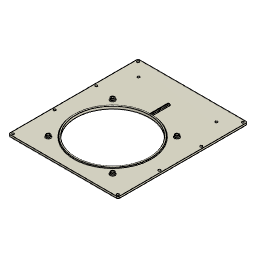
Lid - 120mm Fan (Autodesk Fusion 360 design; units mm, degrees)
Autodesk Fusion 360 part; units mm, degrees
imported_body "Derived Base Feature5" makes body 1
imported_body "Derived Base Feature6" makes body 2
imported_body "Derived Base Feature2" makes body 3
imported_body "Derived Base Feature3" makes body 4
imported_body "Derived Base Feature4" makes body 5
ref_plane "WorkPlane1" through (0, 0, 123.8) normal (0, 0, 1) x (1, 0, 0)
sketch "Sketch1" plane through (0, 0, 123.8) normal (0, 0, 1) x (1, 0, 0)
  circle A0 centre (-85.5, 170) radius 1.4 construction
  line L0 (-81.5, 4) -> (-81.5, 166) construction
  line L1 (-81.5, 166) -> (-81.5, 167) construction
  line L2 (-81.5, 167) -> (-77.5, 167) construction
  line L3 (-77.5, 167) -> (-77.5, 174) construction
  line L4 (-77.5, 174) -> (-81.5, 174) construction
  line L5 (-81.5, 174) -> (-86.5, 174) construction
  line L6 (-87.2574, 174) -> (-87.5, 174) construction
  line L7 (-87.5, 174) -> (-89.5, 172) construction
  line L8 (-89.5, 172) -> (-89.5, 0) construction
  line L9 (-89.5, 0) -> (-81.5, 0) construction
  line L10 (-81.5, 0) -> (-81.5, 4) construction
  circle A1 centre (85.5, 170) radius 1.4 construction
  line L11 (89.5, 0) -> (89.5, 172) construction
  line L12 (89.5, 172) -> (87.5, 174) construction
  line L13 (87.5, 174) -> (86.5, 174) construction
  line L14 (86.5, 174) -> (86.5, 177) construction
  line L15 (86.5, 177) -> (86.45, 177) construction
  line L16 (86.45, 177) -> (86.45, 174) construction
  line L17 (86.45, 174) -> (81.5, 174) construction
  line L18 (81.5, 174) -> (77.5, 174) construction
  line L19 (77.5, 174) -> (77.5, 167) construction
  line L20 (77.5, 167) -> (81.5, 167) construction
  line L21 (81.5, 167) -> (81.5, 0) construction
  line L22 (81.5, 0) -> (89.5, 0) construction
  line L23 (81.5, 0) -> (81.5, -37.7937) construction
  line L24 (81.5, -37.7937) -> (87.5, -37.7937) construction
  line L25 (87.5, -37.7937) -> (89.5, -35.7937) construction
  line L26 (89.5, -35.7937) -> (89.5, -5) construction
  line L27 (89.5, -5) -> (89.5, 0) construction
  line L28 (89.5, 0) -> (81.5, 0) construction
  line L29 (-89.5, 0) -> (-89.5, -35.7937) construction
  line L30 (-89.5, -35.7937) -> (-87.5, -37.7937) construction
  line L31 (-87.5, -37.7937) -> (-81.5, -37.7937) construction
  line L32 (-81.5, -37.7937) -> (-81.5, -5) construction
  line L33 (-81.5, -5) -> (-81.5, 0) construction
  line L34 (-81.5, 0) -> (-89.5, 0) construction
  line L35 (87.5, -37.7937) -> (-87.5, -37.7937) construction
  line L36 (-77.3, 174) -> (77.3, 174) construction
  line L37 (-77.5, 174) -> (77.5, 174)
  line L38 (77.5, 174) -> (87.5, 174)
  line L39 (87.5, 174) -> (89.5, 172)
  line L40 (89.5, 172) -> (89.5, -35.7937)
  line L41 (89.5, -35.7937) -> (87.5, -37.7937)
  line L42 (-87.5, -37.7937) -> (87.5, -37.7937)
  line L43 (-87.5, -37.7937) -> (-89.5, -35.7937)
  line L44 (-89.5, -35.7937) -> (-89.5, 172)
  line L45 (-89.5, 172) -> (-87.5, 174)
  line L46 (-87.5, 174) -> (-77.3, 174)
  circle A2 centre (-85.5, 170) radius 1.8
  circle A3 centre (-85.5, 102) radius 1.8
  circle A4 centre (-85.5, 34) radius 1.8
  circle A5 centre (-85.5, -34) radius 1.8
  circle A6 centre (85.5, -34) radius 1.8
  circle A7 centre (85.5, 34) radius 1.8
  circle A8 centre (85.5, 102) radius 1.8
  circle A9 centre (85.5, 170) radius 1.8
  circle A10 centre (-85.5, -34) radius 1.4 construction
  circle A11 centre (85.5, -34) radius 1.4 construction
  circle A12 centre (85.5, 34) radius 1.4 construction
  circle A13 centre (-85.5, 34) radius 1.4 construction
  circle A14 centre (85.5, 102) radius 1.4 construction
  circle A15 centre (-85.5, 102) radius 1.4 construction
  line L47 (-86.5, 174) -> (-87.2574, 174)
  line L48 (-77.5, 173.8) -> (-77.3, 173.8)
  line L49 (-77.3, 173.8) -> (77.5, 173.8)
  line L50 (77.5, 173.8) -> (87.4172, 173.8)
  line L51 (87.4172, 173.8) -> (89.3, 171.9172)
  line L52 (89.3, 171.9172) -> (89.3, -35.7109)
  line L53 (89.3, -35.7109) -> (87.4172, -37.5937)
  line L54 (-87.4172, -37.5937) -> (87.4172, -37.5937)
  line L55 (-87.4172, -37.5937) -> (-89.3, -35.7109)
  line L56 (-89.3, -35.7109) -> (-89.3, 171.9172)
  line L57 (-89.3, 171.9172) -> (-87.4172, 173.8)
  line L58 (-87.4172, 173.8) -> (-77.3, 173.8)
  dimension "d2" = 0.2
  dimension "d4" = 3.6
  dimension "d5" = 3.6
  dimension "d6" = 3.6
  dimension "d7" = 3.6
  dimension "d8" = 3.6
  dimension "d9" = 3.6
  dimension "d10" = 3.6
  dimension "d11" = 3.6
  constraint coincident L3.end L4.start
  constraint coincident L18.end L19.start
  constraint coincident L12.end L13.start
  constraint coincident L11.end L12.start
  constraint coincident L25.end L26.start
  constraint coincident L24.end L25.start
  constraint coincident L30.end L31.start
  constraint coincident L29.end L30.start
  constraint coincident L7.end L8.start
  constraint coincident L6.end L7.start
  constraint coincident L36.start L46.end
  constraint concentric A0 A2
  constraint concentric A1 A9
  constraint concentric A5 A10
  constraint concentric A6 A11
  constraint concentric A4 A13
  constraint concentric A7 A12
  constraint concentric A8 A14
  constraint concentric A3 A15
  measures "d4" diameter of A2
  measures "d5" diameter of A9
  measures "d6" diameter of A8
  measures "d7" diameter of A3
  measures "d8" diameter of A7
  measures "d9" diameter of A6
  measures "d10" diameter of A4
  measures "d11" diameter of A5
extrude "Extrude1" add sketch "Sketch1" along normal blind 3 separate body contours L48 L49 L50 L51 L52 L53 L54 L55 L56 L57 L58 makes body 6
ref_plane "WorkPlane2" through (-3.8893, 68.1031, 125.3) normal (1, 0, 0) x (0, 1, 0)
sketch "Sketch2" plane through (-3.8893, 68.1031, 125.3) normal (1, 0, 0) x (0, 1, 0)
  line L0 (-105.6969, 1.5) -> (-105.6969, -1.5) construction
  line L1 (-105.6969, -1.5) -> (105.6969, -1.5) construction
  line L2 (105.6969, -1.5) -> (105.6969, 1.5) construction
  line L3 (105.6969, 1.5) -> (-105.6969, 1.5) construction
  line L4 (105.6969, 1.5) -> (65.6969, 1.5) construction
  dimension "d14" = 40
  constraint coincident L2.end L3.start
  constraint perpendicular L2 L4
  measures "d14" distance of L2.end L4.end
ref_plane "WorkPlane3" through (0, -37.5937, 125.3) normal (0, -1, 0) x (1, 0, 0)
sketch "Sketch3" plane through (0, -37.5937, 125.3) normal (0, -1, 0) x (1, 0, 0)
  line L0 (-87.4172, -1.5) -> (87.4172, -1.5)
  line L1 (87.4172, -1.5) -> (87.4172, 1.5)
  line L2 (87.4172, 1.5) -> (-87.4172, 1.5)
  line L3 (-87.4172, 1.5) -> (-87.4172, -1.5)
  line L4 (0, 1.5) -> (0, 26.5) construction
  line L5 (0, 26.5) -> (-45, 26.5)
  line L6 (0, 16.5) -> (-46.4175, 16.5)
  line L7 (-46.4175, 16.5) -> (-56.9175, 1.5)
  line L8 (-45, 26.5) -> (-52.5, 26.5)
  line L9 (-52.5, 26.5) -> (-70, 1.5)
  line L10 (0, 26.5) -> (45, 26.5)
  line L11 (45, 26.5) -> (52.5, 26.5)
  line L12 (52.5, 26.5) -> (70, 1.5)
  line L13 (46.4175, 16.5) -> (56.9175, 1.5)
  line L14 (0, 16.5) -> (46.4175, 16.5)
  dimension "d16" = 25
  constraint midpoint L2 L4.start
  constraint perpendicular L2 L4
  constraint parallel L2 L8
  constraint parallel L7 L9
  constraint coincident L2 L7.end
  constraint coincident L2 L9.end
  constraint symmetric L4 L5.start L10.start
  constraint symmetric L4 L5.end L10.end
  constraint symmetric L4 L9.end L12.end
  constraint symmetric L4 L6.end L13.start
  constraint symmetric L4 L6.start L14.start
  constraint symmetric L4 L8.end L11.end
  constraint symmetric L4 L7.end L13.end
  measures "d16" distance of L4.start L4.end
copy_body "Body->Comp1" bodies 6 removing the originals makes body 7 in component "Lid - Fan and Handle"
sketch "Sketch4" plane through (0, 0, 126.8) normal (0, 0, 1) x (-1, 0, 0)
  circle A0 centre (-85.5, 34) radius 1.8
  circle A1 centre (85.5, -170) radius 1.8
  circle A2 centre (85.5, 34) radius 1.8
  circle A3 centre (-85.5, -170) radius 1.8
  line L0 (87.4172, 37.5937) -> (-87.4172, 37.5937)
  line L1 (-87.4172, 37.5937) -> (-89.3, 35.7109)
  line L2 (-89.3, 35.7109) -> (-89.3, -171.9172)
  line L3 (-89.3, -171.9172) -> (-87.4172, -173.8)
  line L4 (-87.4172, -173.8) -> (-77.5, -173.8)
  line L5 (-77.5, -173.8) -> (77.3, -173.8)
  line L6 (77.3, -173.8) -> (87.4172, -173.8)
  line L7 (87.4172, -173.8) -> (89.3, -171.9172)
  line L8 (89.3, -171.9172) -> (89.3, 35.7109)
  line L9 (89.3, 35.7109) -> (87.4172, 37.5937)
  line L10 (-59.3588, 7.5937) -> (-56.9175, 5.5937)
  line L11 (-56.9175, 5.5937) -> (-56.9175, -10.4063)
  line L12 (-56.9175, -10.4063) -> (-59.3588, -12.4063)
  line L13 (-59.3588, -12.4063) -> (-67.5587, -12.4063)
  line L14 (-67.5587, -12.4063) -> (-70, -10.4063)
  line L15 (-70, -10.4063) -> (-70, 5.5937)
  line L16 (-70, 5.5937) -> (-67.5587, 7.5937)
  line L17 (-67.5587, 7.5937) -> (-59.3588, 7.5937)
  line L18 (56.9175, 5.5937) -> (59.3588, 7.5937)
  line L19 (59.3588, 7.5937) -> (67.5587, 7.5937)
  line L20 (67.5587, 7.5937) -> (70, 5.5937)
  line L21 (70, 5.5937) -> (70, -10.4063)
  line L22 (70, -10.4063) -> (67.5587, -12.4063)
  line L23 (67.5587, -12.4063) -> (59.3588, -12.4063)
  line L24 (59.3588, -12.4063) -> (56.9175, -10.4063)
  line L25 (56.9175, -10.4063) -> (56.9175, 5.5937)
  line L26 (56.9175, -2.4063) -> (70, -2.4063) construction
  line L27 (63.4588, -12.4063) -> (63.4588, 7.5937) construction
  circle A4 centre (63.4588, -2.4063) radius 1.425
  line L28 (0, 0) -> (0, -20) construction
  circle A5 centre (-63.4588, -2.4063) radius 1.425
  circle A6 centre (85.5, -34) radius 1.8
  circle A7 centre (-85.5, -102) radius 1.8
  circle A8 centre (-85.5, -34) radius 1.8
  circle A9 centre (85.5, -102) radius 1.8
  dimension "d30" = 2.85
  constraint midpoint L25 L26.start
  constraint midpoint L21 L26.end
  constraint midpoint L23 L27.start
  constraint midpoint L19 L27.end
  constraint midpoint L26 A4.centre
  constraint coincident L28.start origin
  constraint vertical L28
  constraint symmetric A4 L28 A5
  measures "d30" diameter of A4
sketch "Sketch5" plane through (0, 0, 126.8) normal (0, 0, 1) x (-1, 0, 0)
  circle A0 centre (-85.5, 34) radius 1.8
  circle A1 centre (85.5, -170) radius 1.8
  circle A2 centre (85.5, 34) radius 1.8
  circle A3 centre (-85.5, -170) radius 1.8
  line L0 (87.4172, 37.5937) -> (-87.4172, 37.5937)
  line L1 (-87.4172, 37.5937) -> (-89.3, 35.7109)
  line L2 (-89.3, 35.7109) -> (-89.3, -171.9172)
  line L3 (-89.3, -171.9172) -> (-87.4172, -173.8)
  line L4 (-87.4172, -173.8) -> (-77.5, -173.8)
  line L5 (-77.5, -173.8) -> (77.3, -173.8)
  line L6 (77.3, -173.8) -> (87.4172, -173.8)
  line L7 (87.4172, -173.8) -> (89.3, -171.9172)
  line L8 (89.3, -171.9172) -> (89.3, 35.7109)
  line L9 (89.3, 35.7109) -> (87.4172, 37.5937)
  circle A4 centre (63.4588, -2.4063) radius 1.425 construction
  circle A5 centre (-63.4588, -2.4063) radius 1.425 construction
  line L10 (-63.4588, -148.8) -> (-63.4588, -2.4063) construction
  circle A6 centre (63.4412, -148.8) radius 1.8
  circle A7 centre (-63.4588, -148.8) radius 1.8
  circle A8 centre (85.5, -34) radius 1.8
  circle A9 centre (-85.5, -102) radius 1.8
  circle A10 centre (-85.5, -34) radius 1.8
  circle A11 centre (85.5, -102) radius 1.8
  line L11 (-0.0088, -133.8) -> (-0.0088, -2.4063) construction
  line L12 (52.4912, 9.4861) -> (-52.5088, 9.4861) construction
  line L13 (-52.5088, 9.4861) -> (-52.5088, -95.5139) construction
  line L14 (-52.5088, -95.5139) -> (52.4912, -95.5139) construction
  line L15 (52.4912, -95.5139) -> (52.4912, 9.4861) construction
  line L16 (52.4912, 9.4861) -> (-52.5088, -95.5139) construction
  line L17 (-52.5088, 9.4861) -> (52.4912, -95.5139) construction
  circle A12 centre (-0.0088, -43.0139) radius 60
  circle A13 centre (-52.5088, -95.5139) radius 1.9
  circle A14 centre (52.4912, -95.5139) radius 1.9
  circle A15 centre (52.4912, 9.4861) radius 1.9
  circle A16 centre (-52.5088, 9.4861) radius 1.9
  circle A17 centre (-0.0088, -43.0139) radius 62
  line L18 (-0.0088, -105.0139) -> (-0.0088, -133.8) construction
  line L19 (-1.5088, -104.9957) -> (-1.5088, -133.8)
  line L20 (1.4912, -104.9957) -> (1.4912, -133.8)
  arc A18 (-1.5088, -133.8) -> (1.4912, -133.8) centre (-0.0088, -133.8) ccw
  circle A19 centre (-52.5088, 9.4861) radius 3.1
  circle A20 centre (52.4912, 9.4861) radius 3.1
  circle A21 centre (52.4912, -95.5139) radius 3.1
  circle A22 centre (-52.5088, -95.5139) radius 3.1
  point P0 (-0.0088, -43.0139)
  dimension "d37" = 3.6
  dimension "d38" = 3.6
  dimension "d46" = 126.9
  dimension "d47" = 105
  dimension "d48" = 105
  dimension "d49" = 120
  dimension "d50" = 3.8
  dimension "d51" = 3.8
  dimension "d52" = 3.8
  dimension "d53" = 3.8
  dimension "d54" = 2
  dimension "d57" = 1.2
  dimension "d58" = 1.2
  dimension "d59" = 1.2
  dimension "d60" = 1.2
  constraint coincident A5.centre L10.end
  constraint symmetric A6 A7 L11
  constraint coincident L10.start A7.centre
  constraint horizontal L12
  constraint perpendicular L12 L13
  constraint parallel L12 L14
  constraint parallel L13 L15
  constraint coincident L16 P0
  constraint coincident L17 P0
  constraint coincident L11 P0
  constraint coincident P0 A12.centre
  constraint coincident L13.end L14.start
  constraint coincident L14.end L15.start
  constraint coincident L12.start L15.end
  constraint coincident L12.end L13.start
  constraint coincident A17 L18.start
  constraint coincident L11 L18.start
  constraint tangent L20 A18
  constraint tangent L19 A18
  constraint coincident A17 L19.start
  constraint coincident A17 L20.start
  measures "d37" diameter of A6
  measures "d38" diameter of A7
  measures "d46" distance of A6.centre L10.start
  measures "d47" distance of L13.end L14.end
  measures "d48" distance of L12.end L13.end
  measures "d49" diameter of A12
  measures "d50" diameter of A13
  measures "d51" diameter of A14
  measures "d52" diameter of A15
  measures "d53" diameter of A16
extrude "Extrude4" add sketch "Sketch5" along normal blind 3 contours A19 | A20 | A21 | A22 bodies 7 in component "Lid - Fan and Handle"
extrude "Extrude5" add sketch "Sketch5" along normal blind 2 contours A17 | A17 L19 L20 A18 bodies 7 in component "Lid - Fan and Handle"
extrude "Extrude2" cut sketch "Sketch5" against normal blind 3 contours A12 | A13 | A14 | A15 | A16 bodies 7 in component "Lid - Fan and Handle"
fillet "Fillet2" radius 1 1 faces at (-0.4912, 124.1986, 128.8) on bodies 7 in component "Lid - Fan and Handle"
fillet "Fillet3" radius 1 8 edges at (0.0088, -18.9861, 126.8) (-1.4912, 119.3979, 126.8) (0.0088, 135.3, 126.8) (1.5088, 119.3979, 126.8) (-49.601, 94.3929, 126.8) (55.399, 94.3929, 126.8) (55.399, -10.6071, 126.8) (-49.601, -10.6071, 126.8) on bodies 7 in component "Lid - Fan and Handle"
delete_body "RemoveBody2" bodies 3
delete_body "RemoveBody3" bodies 1
delete_body "RemoveBody4" bodies 2
delete_body "RemoveBody5" bodies 4
delete_body "RemoveBody6" bodies 5
copy_body "CopyPasteBodies1" bodies 7 makes body 8 in component "Lid - Fan Only"
move_body "Move1" bodies 8 to x (1, 0, 0) y (0, 1, 0) z (0, 0, 1) at (0, 0, 0) in component "Lid - Fan Only"
extrude "Extrude6" cut sketch "Sketch5" against normal blind 3 contours A6 | A7 bodies 7 in component "Lid - Fan and Handle"
component "Lid - Fan and Handle" placed x (1, 0, 0) y (0, 1, 0) z (0, 0, 1) at (0, 0, 0)
component "Lid - Fan Only" placed x (1, 0, 0) y (0, 1, 0) z (0, 0, 1) at (0, 0, 0)
equation "large_m3 = 3.6 mm"
equation "d4 = large_m3"
equation "d5 = d4"
equation "d6 = d4"
equation "d7 = d4"
equation "d8 = d4"
equation "d9 = d4"
equation "d10 = d4"
equation "d11 = d4"
named bodies: "Body1 (Context1)", "Body1 (1) (Context1)", "Body1 (2) (Context1)", "Body1 (Context2)", "Body1 (1) (Context2)"
